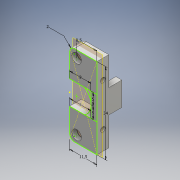
# Autodesk Inventor part: togh
Saved by Autodesk Inventor 2016 (Build 200138000, 138)
## iProperties
Created: 2017-05-26
Part Number: togh
Material: ABS Plastic
Document SubType Name: Modeling
Designer: Karol
Density: 1.06 g/cm^3
Appearance: Smooth - White
Author: Karol
Autodesk Inventor part; units mm, degrees
ref_plane "YZ Plane" through (0, 0, 0) normal (1, 0, 0) x (0, 1, 0)
ref_plane "XZ Plane" through (0, 0, 0) normal (0, 1, 0) x (-1, 0, 0)
ref_plane "XY Plane" through (0, 0, 0) normal (0, 0, 1) x (1, 0, 0)
sketch "Sketch1" plane through (0, 0, 0) normal (0, 1, 0) x (-1, 0, 0)
  line L0 (3.75, 17) -> (-5.75, 17)
  line L1 (-5.75, 17) -> (-5.75, -17)
  line L2 (-5.75, -17) -> (3.75, -17)
  line L3 (5.75, 17) -> (-5.75, -17) construction
  line L4 (-5.75, 17) -> (5.75, -17) construction
  arc A0 (5.75, 15) -> (3.75, 17) centre (3.75, 15) ccw
  arc A1 (3.75, -17) -> (5.75, -15) centre (3.75, -15) ccw
  line L5 (-3.25, 0) -> (-3.25, 5)
  line L6 (-3.25, 0) -> (-3.25, -5)
  line L7 (-3.25, -5) -> (5.75, -5)
  line L8 (-3.25, 5) -> (5.75, 5)
  line L9 (5.75, 5) -> (5.75, 15)
  line L10 (5.75, -5) -> (5.75, -15)
  arc A2 (-0.5666, 5) -> (-0.5666, -5) centre (2.75, 0) ccw
  line L11 (-3.25, 5) -> (-5.75, 5)
  line L12 (-3.25, -5) -> (-5.75, -5)
  point P0 (2.75, 14)
  point P1 (2.75, -14)
  dimension "d0" = 11.5
  dimension "d1" = 34
  dimension "d2" = 2
  dimension "d29" = 5
  dimension "d30" = 5
  dimension "d31" = 9
  dimension "d32" = 9
  dimension "d48" = 8.5
  constraints: 26 end point, 6 point on circle, 6 point on line, 4 vertical, 3 centre point, 3 horizontal, 2 parallel, 2 perpendicular, 2 tangent, 1 coincident, 1 equal radius
  measures "d0" distance of L4.end L1.end
  measures "d1" distance of L1.end L0.end
  measures "d2" radius of A0
  measures "d29" distance of L5.start L5.end
  measures "d30" distance of L5.start L6.end
  measures "d31" distance of L6.end L7.end
  measures "d32" distance of L5.end L8.end
  measures "d48" distance from line of L1 point (2.75, 14)
extrude "Extrusion1" add sketch "Sketch1" along normal blind 5 contours A0 L9 L8 L11 L1 L0 | L11 L5 L6 L12 L1 | L12 L7 L10 A1 L2 L1
hole "Hole1" at (-2.75, 0, 14) at (-2.75, 0, -14) direction (0, 1, 0) diameter 3.5 depth 8
sketch "Sketch5" plane through (-5.75, 0, 5) normal (-1, 0, 0) x (0, 0, 1)
  point P0 (-5, 0)
  point P1 (4, 2.5)
  point P2 (-14, 2.5)
hole "Hole3" at (-5.75, 2.5, 9) at (-5.75, 2.5, -9) direction (1, 0, 0) diameter 2 depth 12
extrude "Extrusion4" add sketch "Sketch1" along normal blind 10.5 contours L11 L5 L6 L12 L1
ref_plane "Work Plane4" through (0, 2, 0) normal (0, -1, 0) x (1, 0, 0)
sketch "Sketch9" plane through (0, 2, 0) normal (0, -1, 0) x (1, 0, 0)
  circle A0 centre (-2.75, -14) radius 1.75 projected
  circle A1 centre (-2.75, 14) radius 1.75 projected
  circle A2 centre (-2.75, 14) radius 2
  circle A3 centre (-2.75, -14) radius 2
  point P0 (0, 0)
  dimension "d61" = 4
  dimension "d62" = 4
  constraints: 2 centre point, 2 coincident
  measures "d61" diameter of A2
  measures "d62" diameter of A3
extrude "Extrusion7" cut sketch "Sketch9" along normal blind 10
body "Solid1"
